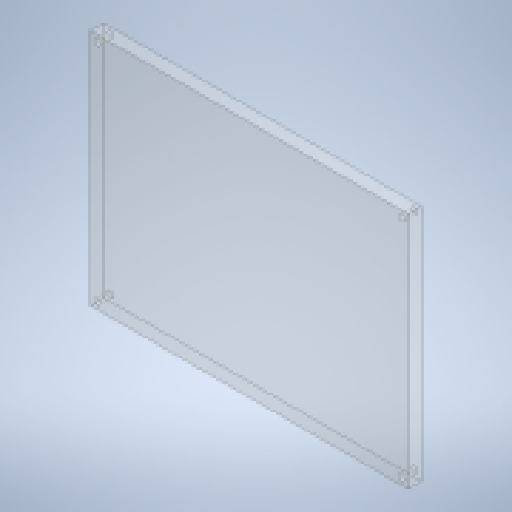
# Autodesk Inventor part: chest_box_cap
Saved by Autodesk Inventor 2024 (Build 280153000, 153)
## iProperties
Created: 2024-09-18
Part Number: chest_box_cap
Material: PMMA 플라스틱
Document SubType Name: Modeling
Designer: Eungang
Density: 1.188 g/cm^3
Appearance: 폴리카보네이트 - 선명
Author: Eungang
Autodesk Inventor part; units mm, degrees
ref_plane "YZ Plane" through (0, 0, 0) normal (1, 0, 0) x (0, 1, 0)
ref_plane "XZ Plane" through (0, 0, 0) normal (0, 1, 0) x (-1, 0, 0)
ref_plane "XY Plane" through (0, 0, 0) normal (0, 0, 1) x (1, 0, 0)
sketch "스케치1" plane through (0, 0, 0) normal (0, 0, 1) x (1, 0, 0)
  line L0 (-155, 119.2) -> (0, 119.2) projected
  line L1 (-155, 0) -> (-155, 119.2) projected
  line L2 (0, 0) -> (-155, 0) projected
  line L3 (0, 119.2) -> (0, 0) projected
  line L4 (-6.2, 113) -> (-148.8, 113)
  line L5 (-148.8, 113) -> (-148.8, 6.2)
  line L6 (-148.8, 6.2) -> (-6.2, 6.2)
  line L7 (-6.2, 6.2) -> (-6.2, 113)
  circle A0 centre (-9.2, 110) radius 1.35 projected
  circle A1 centre (-145.8, 110) radius 1.35 projected
  circle A2 centre (-145.8, 9.2) radius 1.35 projected
  circle A3 centre (-9.2, 9.2) radius 1.35 projected
  point P0 (-6, 113.2)
  constraints: 8 end point
extrude "돌출1" add sketch "스케치1" against normal blind 6 contours L7 L6 L5 L4
